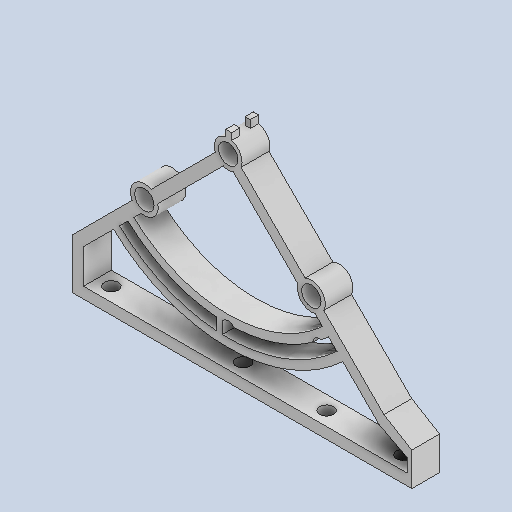
# Autodesk Inventor part: BigCageP2
Saved by Autodesk Inventor 2025 (Build 290162000, 162)
## iProperties
Created: 2025-08-07
Part Number: BigCageP2
Material: Generic
Document SubType Name: Modeling
Designer: Pravoslav
Density: 1 g/cm^3
Appearance: Default
Author: Pravoslav
Autodesk Inventor part; units mm, degrees
ref_plane "YZ Plane" through (0, 0, 0) normal (1, 0, 0) x (0, 1, 0)
ref_plane "XZ Plane" through (0, 0, 0) normal (0, 1, 0) x (-1, 0, 0)
ref_plane "XY Plane" through (0, 0, 0) normal (0, 0, 1) x (1, 0, 0)
sketch "Sketch1" plane through (0, 0, 0) normal (0, 0, 1) x (1, 0, 0)
  line L0 (-70, 2) -> (70, 2)
  line L1 (70, 2) -> (70, -2)
  line L2 (70, -2) -> (-70, -2)
  line L3 (-70, -2) -> (-70, 2)
  line L4 (-70, 2) -> (70, -2) construction
  line L5 (70, 2) -> (-70, -2) construction
  line L6 (-70, 2) -> (44.4369, 116.4369)
  line L7 (-70, 2) -> (91.8383, 2) construction
  line L8 (70, 2) -> (-21.2026, 93.2026)
  line L9 (-64.3431, 2) -> (2.8284, 69.1716)
  line L10 (-2.8284, 69.1716) -> (64.3431, 2)
  circle A0 centre (0, 69.1716) radius 3.5
  circle A1 centre (0, 69.1716) radius 5
  circle A2 centre (-67.6199, 0) radius 3.5
  circle A3 centre (-67.6199, 0) radius 5
  circle A4 centre (69.5355, 2.4645) radius 3.5
  circle A5 centre (69.5355, 2.4645) radius 5
  circle A6 centre (29.8984, 39.897) radius 3.5
  circle A7 centre (29.8984, 39.897) radius 5
  line L11 (27.6414, 44.3586) -> (-27.6414, 44.3586)
  line L12 (-27.6414, 44.3586) -> (-27.6414, 52.2202)
  line L13 (-27.6414, 52.2202) -> (-24.6414, 52.2202)
  line L14 (-24.6414, 52.2202) -> (-24.6414, 47.3586)
  line L15 (27.6414, 44.3586) -> (27.6414, 52.2202)
  line L16 (27.6414, 52.2202) -> (24.6414, 52.2202)
  line L17 (24.6414, 52.2202) -> (24.6414, 47.3586)
  circle A8 centre (0, 69.1716) radius 50
  circle A9 centre (0, 69.1716) radius 53
  circle A10 centre (0, 69.1716) radius 57.3
  circle A11 centre (0, 69.1716) radius 60.3
  arc A12 (2.1548, 16.1686) -> (-2.1058, 16.2485) centre (-0.005, 14.6373) ccw
  arc A13 (33.4747, 28.0809) -> (30.3172, 25.699) centre (32.9561, 25.4847) ccw
  line L18 (-2.1058, 16.2485) -> (-2.1315, 16.2145)
  line L19 (-0.1162, 2) -> (-0.1162, -3.5)
  circle A14 centre (-30.1308, 39.897) radius 3.5
  circle A15 centre (-30.1308, 39.897) radius 5
  line L20 (-70.2324, 2) -> (69.7676, -2) construction
  circle A16 centre (-30.1308, 39.897) radius 3.5
  circle A17 centre (-30.1308, 39.897) radius 5
  line L21 (-56, -2) -> (-56, 16)
  line L22 (-52, 20) -> (-52, -2)
  line L23 (-2.1315, 16.2145) -> (-2.1315, 11.9112)
  line L24 (-4.1487, 16.3342) -> (-4.1487, 12.022)
  line L25 (64.3431, 2) -> (64.3431, -2)
  line L26 (66, -2) -> (66, 13.8793)
  line L27 (66, 10) -> (55.978, 16.022)
  line L28 (66, 6) -> (54.3212, 12.022)
  line L29 (64.3431, 2) -> (64.3431, 6.8543)
  point P0 (0, 0)
  point P1 (1.8262, 64.517)
  point P2 (25.0868, 41.2564)
  point P3 (31.2578, 35.0853)
  point P4 (64.3431, 2)
  point P5 (-1.8262, 64.517)
  point P6 (-4.6546, 67.3454)
  point P7 (-67.0344, 4.9656)
  point P8 (-63.0374, -2)
  point P9 (67.2842, -2)
  point P10 (66, 6)
  point P11 (34.36, 37.64)
  point P12 (4.6546, 67.3454)
  point P13 (-41.2009, 25.1423)
  point P14 (41.2009, 25.1423)
  point P15 (39.0783, 27.2648)
  point P16 (-39.0783, 27.2648)
  point P17 (-36.0358, 30.3074)
  point P18 (36.0358, 30.3074)
  point P19 (33.9128, 32.4303)
  point P20 (-33.9128, 32.4303)
  point P21 (2.1218, 16.2141)
  point P22 (-31.3061, 35.0371)
  point P23 (-25.2709, 41.0722)
  point P24 (-27.7217, 44.2783)
  point P25 (-34.5122, 37.4878)
  point P26 (-56, 7)
  point P27 (-52, 2)
  point P28 (-52, 14.3431)
  point P29 (-56, 10.3431)
  point P30 (-56, 2)
  point P31 (44.0293, 27.9707)
  point P32 (41.2009, 113.2009)
  point P33 (1.8262, 73.8262)
  point P34 (0, 66.3431)
  point P35 (0, 72)
  point P36 (21.9846, 44.3586)
  point P37 (63.9523, 2.3909)
  point P38 (-21.9846, 44.3586)
  point P39 (64.5572, 2)
  point P40 (-1.8262, 73.8262)
  point P41 (-44.0293, 27.9707)
  point P42 (70, -1.78)
  point P43 (-26.636, 39.7071)
  point P44 (-29.941, 36.4021)
  point P45 (36.7413, 35.2587)
  point P46 (38.8642, 33.1358)
  point P47 (41.9067, 30.0933)
  point P48 (64.3431, 2)
  dimension "d14" = 10
  dimension "d16" = 10
  dimension "d0" = 140
  dimension "d1" = 4
  dimension "d2" = 45
  dimension "d3" = 4
  dimension "d6" = 4
  dimension "d7" = 4
  dimension "d8" = 4
  dimension "d9" = 7
  dimension "d10" = 10
  dimension "d11" = 7
  dimension "d12" = 10
  dimension "d13" = 7
  dimension "d15" = 7
  dimension "d17" = 3
  dimension "d18" = 3
  dimension "d21" = 3
  dimension "d22" = 3
  dimension "d23" = 4.3
  dimension "d24" = 100
  dimension "d42" = 4
  dimension "d43" = 14
  dimension "d62" = 4
  dimension "d63" = 4
  dimension "d64" = 4
  dimension "d65" = 8
  constraints: 60 end point, 23 point on line, 16 centre point, 10 coincident, 10 perpendicular, 10 point on circle, 6 symmetric about line, 4 parallel, 3 horizontal, 3 midpoint, 3 vertical, 1 equal length, 10 other
  measures "d0" distance of L1.end L2.end
  measures "d1" distance between parallel lines of L0 L2
  measures "d2" angle of L7 L6
  measures "d3" distance from line of L9.end L6
  measures "d6" distance from line of L6 L9.start
  measures "d7" distance from line of L10.start L8
  measures "d8" distance from line of L10 L0.end
  measures "d9" diameter of A0
  measures "d10" diameter of A1
  measures "d11" diameter of A2
  measures "d12" diameter of A3
  measures "d13" diameter of A4
  measures "d15" diameter of A6
  measures "d17" distance of L12.end L13.end
  measures "d18" distance of L15.end L16.end
  measures "d21" radial gap between concentric circles of A9 A8
  measures "d22" radial gap between concentric circles of A11 A10
  measures "d23" radial gap between concentric circles of A9 A10
  measures "d24" diameter of A8
  measures "d42" distance from line of point (-56, 7) L22
  measures "d43" distance between parallel lines of L3 L21
  measures "d62" distance between parallel lines of L1 L26
  measures "d63" vertical distance of L27.end L28.end
  measures "d64" distance of L27.start L28.start
  measures "d65" distance from line of L2 L28.start
extrude "Extrusion1" add sketch "Sketch1" along normal blind 10 contours L19 L2 L22 L0 | L0 L25 L2 L19 | L29 L28 A5 L0 | L0 A5 L26 L2 L25 | L22 L2 L21 L0 | L0 L21 L9 L22 | A5 L26 L0 | L0 L26 A5 | L10 A11 L8 L28 | L22 L6 A11 L9 | L9 L21 L6 L22 | L8 L27 L26 | A11 L9 A10 L10 | L10 A10 L8 A11 | A11 L6 A10 L9 | L10 A9 L8 A10 | A10 L6 A9 L9 | A9 A13 A12 L18 L9 A8 L10 | L10 A8 L8 A9 | A10 L24 A9 L23 | A9 L6 A8 L9 | L10 A7 L8 A8 | A8 L6 A15 L9 | A7 L10 A6 | L10 A6 L8 A7 | A15 L6 A14 L9 | L9 A14 A15 | A7 L8 A6 L10 | L10 L11 A7 | L8 A6 A7 | A15 L6 A14 | L10 A1 L8 L11 | A14 L6 A15 L9 | L6 L11 L9 A15 | A1 L8 A0 L6 | L6 A0 L8 A1 | A1 L9 A0 L10 | L10 A0 L8 A1 | L11 L6 A1 L9 | L8 A0 L6 A1 | A1 L6 A0 L9
extrude "Extrusion2" cut sketch "Sketch1" along normal blind 10 contours A9 A13 | L18 A12 A9
sketch "Sketch3" plane through (-70, -2, 0) normal (0, -1, 0) x (1, 0, 0)
  line L0 (134.3431, 0) -> (134.3431, 10) projected
  line L1 (5.6569, 0) -> (5.6569, 10) projected
  circle A0 centre (23, 5) radius 2.5
  circle A1 centre (128, 5) radius 2.5
  line L2 (140, 0) -> (140, 10) projected
  line L3 (14, 10) -> (136, 10) projected
  point P0 (70, 0)
  point P1 (0, 10)
  point P2 (133.7935, 10)
  point P3 (18, 10)
  dimension "d34" = 5
  dimension "d35" = 5
  dimension "d36" = 105
  dimension "d37" = 12
  dimension "d38" = 5
  dimension "d39" = 5
  constraints: 2 centre point
  measures "d34" diameter of A0
  measures "d35" diameter of A1
  measures "d36" distance of A1.centre A0.centre
  measures "d37" distance from line of L2 A1.centre
  measures "d38" distance from line of L3 A1.centre
  measures "d39" distance from line of L3 A0.centre
extrude "Extrusion4" cut sketch "Sketch3" against normal up to surface (4 mm away)
sketch "Sketch6" plane through (0, 0, 10) normal (0, 0, 1) x (1, 0, 0)
  line L0 (-0.8413, 73.4692) -> (1.2373, 73.4692)
  line L1 (1.2373, 73.4692) -> (1.2373, 76.4217)
  line L2 (1.2373, 76.4217) -> (-0.8413, 76.4217)
  line L3 (-0.8413, 76.4217) -> (-0.8413, 73.4692)
  point P0 (0, 0)
  constraints: 8 end point, 2 parallel, 1 horizontal, 1 perpendicular
extrude "Extrusion7" add sketch "Sketch6" against normal blind 3
sketch "Sketch4" plane through (0, 0, 0) normal (0, 0, -1) x (-1, 0, 0)
  circle A0 centre (0, 69.1716) radius 3.5 projected
  arc A1 (-4.6546, 67.3454) -> (-1.8262, 64.517) centre (0, 69.1716) ccw projected
  line L0 (-0.9508, 73.5061) -> (0.9164, 73.5061)
  line L1 (0.9164, 73.5061) -> (0.9164, 76.8255)
  line L2 (0.9164, 76.8255) -> (-0.9508, 76.8255)
  line L3 (-0.9508, 76.8255) -> (-0.9508, 73.5061)
  point P0 (0, 0)
  point P1 (3.5355, 65.136)
  point P2 (4.6546, 67.3454)
  point P3 (3.5355, 65.636)
  point P4 (3.5355, 65.636)
  point P5 (1.8262, 64.517)
  point P6 (-3.4452, 68.5548)
  point P7 (-0.6168, 65.7263)
  constraints: 8 end point, 2 parallel, 2 point on circle, 1 horizontal, 1 perpendicular
extrude "Extrusion5" add sketch "Sketch4" against normal blind 3 contours L3 L2 L1 L0
sketch "Sketch5" plane through (-56, -2, 0) normal (0, -1, 0) x (1, 0, 0)
  circle A0 centre (56.3685, 5) radius 2.5
  circle A1 centre (86.3685, 5) radius 2.5
  line L0 (0, 10) -> (122, 10) projected
  line L1 (53.8685, 0) -> (53.8685, 10) projected
  point P0 (56, 0)
  point P1 (119.7935, 10)
  point P2 (-14, 10)
  point P3 (126, 10)
  point P4 (4, 10)
  dimension "d52" = 5
  dimension "d53" = 5
  dimension "d54" = 5
  dimension "d55" = 0
  dimension "d56" = 30
  dimension "d57" = 2.5
  constraints: 2 centre point
  measures "d52" diameter of A0
  measures "d53" diameter of A1
  measures "d54" distance from line of L0 A1.centre
  measures "d55" vertical distance of A0.centre A1.centre
  measures "d56" distance of A0.centre A1.centre
  measures "d57" distance from line of L1 A0.centre
extrude "Extrusion6" cut sketch "Sketch5" against normal up to surface (4 mm away)
body "Solid1"
